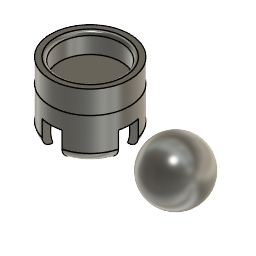
Ball Wheel (old) (Autodesk Fusion 360 design; units mm, degrees)
Autodesk Fusion 360 part; units mm, degrees
sketch "Sketch1" plane through (0, 0, 0) normal (0, 0, 1) x (1, 0, 0)
  circle A0 centre (0, 0) radius 12
  dimension "d2" = 24
  measures "d2" diameter of A0
extrude "Extrude1" add sketch "Sketch1" along normal blind 17 makes body 1
sketch "Sketch2" plane through (0, 0, 17) normal (0, 0, 1) x (-1, 0, 0)
  circle A0 centre (0, 0) radius 12
  circle A1 centre (0, 0) radius 9.375
  dimension "d5" = 18.75
  constraint coincident A0.centre A1.centre
  measures "d5" diameter of A1
extrude "Extrude2" cut sketch "Sketch2" against normal blind 6 contours A1 bodies 1
fillet "Fillet1" radius 1 1 edges at (8.7406, -3.3901, 17) on bodies 1
extrude "Extrude4" cut 1 faces at (1.8223, 1.3289, 0) along direction (0, 0, 1) blind 10 on bodies 1 bodies 1
sphere "SpherePrimitive1" add diameter 19 placed x (1, 0, 0) y (0, 0, -1) z (0, 1, 0) at (0, 0, 0) separate body makes body 2
move_body "MoveFace1" bodies 2 to x (1, 0, 0) y (0, 1, 0) z (0, 0, 1) at (0, 0, 0.5) on bodies 2
extrude "Extrude5" add 1 faces at (1.8223, 1.3289, 10) along direction (0, 0, -1) blind 13 separate body on bodies 1 makes body 3
combine "Combine1" operation cut target body 3 tool bodies 2
sketch "Sketch7" plane through (0, 0, -3) normal (0, 0, -1) x (1, 0, 0)
  circle A0 centre (0, 0) radius 8.8318
  circle A1 centre (0, 0) radius 12
  line L0 (13, -3) -> (-13, -3)
  line L1 (-13, -3) -> (-13, 3)
  line L2 (-13, 3) -> (13, 3)
  line L3 (13, 3) -> (13, -3)
  line L4 (3, -13) -> (-3, -13)
  line L5 (-3, -13) -> (-3, 13)
  line L6 (-3, 13) -> (3, 13)
  line L7 (3, 13) -> (3, -13)
  constraint horizontal L0
  constraint vertical L1
  constraint horizontal L2
  constraint vertical L3
  constraint horizontal L4
  constraint vertical L5
  constraint horizontal L6
  constraint vertical L7
extrude "Extrude6" cut sketch "Sketch7" against normal blind 8 contours A0 A1 L0 L2 | A0 A1 L5 L7 | A0 A1 L5 L7 | A0 A1 L0 L2 bodies 3
fillet "Fillet3" radius 3 4 edges at (-8.4853, -8.4853, -3) (-8.4853, 8.4853, -3) (8.4853, 8.4853, -3) (8.4853, -8.4853, -3) on bodies 3
sphere "SpherePrimitive2" add diameter 18 placed x (1, 0, 0) y (0, 1, 0) z (0, 0, 1) at (0, 0, 0) separate body makes body 4
move_body "MoveFace2" bodies 4 to x (1, 0, 0) y (0, 1, 0) z (0, 0, 1) at (26, 0, 0) on bodies 4
